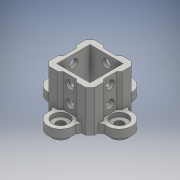
# Autodesk Inventor part: Mat_sup
Saved by Autodesk Inventor 2016 (Build 200138000, 138)
## iProperties
Created: 2016-07-08
Part Number: Mat_sup
Material: Générique
Document SubType Name: Modeling
Designer: LogOut
Density: 1 g/cm^3
Appearance: Par défaut
Author: LogOut
Autodesk Inventor part; units mm, degrees
ref_plane "YZ Plane" through (0, 0, 0) normal (1, 0, 0) x (0, 1, 0)
ref_plane "XZ Plane" through (0, 0, 0) normal (0, 1, 0) x (-1, 0, 0)
sketch "Esquisse1" plane through (0, 0, 0) normal (0, 0, 1) x (1, 0, 0)
  line L0 (-14.142136, 0) -> (0, -14.142136)
  line L1 (0, -14.142136) -> (14.142136, 0)
  line L2 (14.142136, 0) -> (0, 14.142136)
  line L3 (0, 14.142136) -> (-14.142136, 0)
  line L4 (-14.142136, 0) -> (14.142136, 0) construction
  line L5 (0, 14.142136) -> (0, -14.142136) construction
  line L6 (-20.142136, -20.142136) -> (20.142136, -20.142136)
  line L7 (20.142136, -20.142136) -> (20.142136, 20.142136)
  line L8 (20.142136, 20.142136) -> (-20.142136, 20.142136)
  line L9 (-20.142136, 20.142136) -> (-20.142136, -20.142136)
  circle A0 centre (14.142136, 0) radius 6
  circle A1 centre (0, -14.142136) radius 6
  circle A2 centre (-14.142136, 0) radius 6
  circle A3 centre (0, 14.142136) radius 6
  line L10 (0, 19.79899) -> (19.79899, 0)
  line L11 (19.79899, 0) -> (0, -19.79899)
  line L12 (0, -19.79899) -> (-19.79899, 0)
  line L13 (-19.79899, 0) -> (0, 19.79899)
  point P0 (0, 0)
  dimension "d4" = 20
  dimension "d5" = 20
  dimension "d10" = 6
  dimension "d11" = 6
  dimension "d12" = 6
  dimension "d13" = 6
  dimension "d19" = 4
  constraints: 28 end point, 6 parallel, 4 centre point, 4 coincident, 4 tangent, 3 perpendicular, 2 horizontal, 2 midpoint, 3 other
  measures "d4" distance between parallel lines of L0 L2
  measures "d5" distance between parallel lines of L1 L3
  measures "d10" distance from line of L8 L2.end
  measures "d11" distance from line of L9 L0.start
  measures "d12" distance from line of L7 L1.end
  measures "d13" distance from line of L0.end L6
  measures "d19" distance between parallel lines of L2 L10
extrude "Extrusion1" add sketch "Esquisse1" along normal blind 6 contours L3 A2 L0 | L0 A2 L12 L13 L3 | A2 L3 A3 L2 A0 L1 A1 L0 | L0 A1 L12 A2 | A2 L13 A3 L3 | A1 L1 L0 | L0 L1 A1 L11 L12 | A2 L13 L12 | A3 L13 L10 L2 L3 | L3 L2 A3 | L1 A0 L11 A1 | L12 L11 A1 | A3 L10 L13 | A3 L10 A0 L2 | A0 L2 L1 | L1 L2 A0 L10 L11 | L11 L10 A0
sketch "Esquisse2" plane through (0, 0, 0) normal (0, 0, -1) x (-1, 0, 0)
  line L0 (2.828427, 11.313708) -> (11.313708, 2.828427)
  arc A0 (4.242641, 9.899495) -> (-4.242641, 9.899495) centre (0, 14.142136) ccw
  line L1 (-11.313708, 2.828427) -> (-2.828427, 11.313708)
  arc A1 (-9.899495, 4.242641) -> (-9.899495, -4.242641) centre (-14.142136, 0) ccw
  line L2 (-2.828427, -11.313708) -> (-11.313708, -2.828427)
  arc A2 (-4.242641, -9.899495) -> (4.242641, -9.899495) centre (0, -14.142136) ccw
  line L3 (11.313709, -2.828427) -> (2.828427, -11.313708)
  arc A3 (9.899495, -4.242641) -> (9.899495, 4.242641) centre (14.142136, 0) ccw
  circle A4 centre (0, -14.142136) radius 4
  line L4 (-1.035276, -10.278432) -> (-10.278432, -1.035276)
  circle A5 centre (-14.142136, 0) radius 4
  line L5 (-10.278432, 1.035276) -> (-1.035276, 10.278432)
  circle A6 centre (0, 14.142136) radius 4
  line L6 (1.035276, 10.278432) -> (10.278432, 1.035276)
  circle A7 centre (14.142136, 0) radius 4
  line L7 (10.278432, -1.035276) -> (1.035276, -10.278432)
  line L8 (5.795555, -12.589221) -> (12.589221, -5.795555)
  line L9 (-12.589221, -5.795555) -> (-5.795555, -12.589221)
  line L10 (12.589221, 5.795555) -> (5.795555, 12.589221)
  line L11 (-5.795555, 12.589221) -> (-12.589221, 5.795555)
  line L12 (5.990705, -13.808285) -> (13.808285, -5.990705)
  line L13 (-13.808285, -5.990705) -> (-5.990705, -13.808285)
  line L14 (-5.990705, 13.808285) -> (-13.808285, 5.990705)
  line L15 (13.808285, 5.990705) -> (5.990705, 13.808285)
  point P0 (0, 0)
  dimension "d16" = 2
  constraints: 40 point on circle, 32 end point, 11 centre point, 8 point on line
  measures "d16" radial gap between concentric circles of A2 A4
extrude "Extrusion2" cut sketch "Esquisse2" against normal blind 2 contours A6 L1 A0 L0 | L0 A7 L6 A6 | A0 L10 A3 L0 | L6 A7 L7 A4 L4 A5 L5 A6 | A3 L3 A7 L0 | A0 L15 A3 L10 | L5 A5 L1 A6 | A7 L3 A4 L7 | L1 A1 L11 A0 | A0 L11 A1 L14 | A5 L2 A1 L1 | L12 A2 L8 A3 | L4 A4 L2 A5 | A3 L8 A2 L3 | L3 A2 L2 A4 | A1 L9 A2 L13 | L2 A2 L9 A1
sketch "Esquisse3" plane through (0, 0, 6) normal (0, 0, 1) x (1, 0, 0)
  line L0 (-5.990705, 13.808285) -> (-13.808285, 5.990705)
  arc A0 (-13.808285, 5.990705) -> (-13.808285, -5.990705) centre (-14.142136, 0) ccw
  line L1 (-13.808285, -5.990705) -> (-5.990705, -13.808285)
  arc A1 (-5.990705, -13.808285) -> (5.990705, -13.808285) centre (0, -14.142136) ccw
  line L2 (5.990705, -13.808285) -> (13.808285, -5.990705)
  arc A2 (13.808285, -5.990705) -> (13.808285, 5.990705) centre (14.142136, 0) ccw
  line L3 (13.808285, 5.990705) -> (5.990705, 13.808285)
  arc A3 (5.990705, 13.808285) -> (-5.990705, 13.808285) centre (0, 14.142136) ccw
  point P0 (0, 0)
hole "Perçage1" at (-14.142136, 0, 6) at (0, 14.142136, 6) at (14.142136, 0, 6) at (0, -14.142136, 6) direction (0, 0, -1) diameter 4 end through all counterbore diameter 8 counterbore depth 2
sketch "Esquisse4" plane through (0, 0, 6) normal (0, 0, 1) x (1, 0, 0)
  line L0 (-8, -8) -> (8, -8)
  line L1 (8, -8) -> (8, 8)
  line L2 (8, 8) -> (-8, 8)
  line L3 (-8, 8) -> (-8, -8)
  point P0 (0, 0)
  dimension "d27" = 8
  dimension "d28" = 8
  dimension "d29" = 16
  dimension "d33" = 16
  constraints: 8 end point, 2 parallel, 1 horizontal, 1 perpendicular
  measures "d27" distance from line of point (0, 0) L3
  measures "d28" distance from line of point (0, 0) L2
  measures "d29" distance between parallel lines of L3 L1
  measures "d33" distance between parallel lines of L2 L0
extrude "Extrusion3" cut sketch "Esquisse4" against normal through all
sketch "Esquisse5" plane through (0, 0, 6) normal (0, 0, 1) x (1, 0, 0)
  line L0 (8, 8) -> (8, -8)
  line L1 (8, -8) -> (-8, -8)
  line L2 (-8, -8) -> (-8, 8)
  line L3 (-8, 8) -> (8, 8)
  line L4 (-5.990705, 13.808285) -> (-13.808285, 5.990705)
  line L5 (-13.808285, -5.990705) -> (-5.990705, -13.808285)
  line L6 (5.990705, -13.808285) -> (13.808285, -5.990705)
  line L7 (13.808285, 5.990705) -> (5.990705, 13.808285)
  line L8 (-5.990705, 13.808285) -> (-13.808285, 5.990705)
  line L9 (-13.808285, 5.990705) -> (-10.979858, 3.162278)
  arc A0 (-10.979858, -3.162278) -> (-10.979858, 3.162278) centre (-14.142136, 0) ccw
  line L10 (-13.808285, -5.990705) -> (-10.979858, -3.162278)
  line L11 (8, -8) -> (-8, 8) construction
  line L12 (8, 8) -> (-8, -8) construction
  arc A1 (-3.162278, 10.979858) -> (3.162278, 10.979858) centre (0, 14.142136) ccw
  arc A2 (3.162278, -10.979858) -> (-3.162278, -10.979858) centre (0, -14.142136) ccw
  arc A3 (10.979858, 3.162278) -> (10.979858, -3.162278) centre (14.142136, 0) ccw
  line L13 (-5.990705, 13.808285) -> (-3.162278, 10.979858)
  line L14 (5.990705, 13.808285) -> (3.162278, 10.979858)
  line L15 (13.808285, 5.990705) -> (10.979858, 3.162278)
  line L16 (5.990705, -13.808285) -> (3.162278, -10.979858)
  line L17 (-5.990705, -13.808285) -> (-3.162278, -10.979858)
  line L18 (13.808285, -5.990705) -> (10.979858, -3.162278)
  point P0 (0, 0)
  constraints: 36 end point, 8 point on circle, 8 tangent, 4 centre point, 3 symmetric about line, 2 perpendicular, 3 other
extrude "Extrusion4" add sketch "Esquisse5" along normal blind 16
chamfer "Chanfrein1" distance 4 angle 45 8 edges at (-13.8083, 5.9907, 14) (-5.9907, 13.8083, 14) (5.9907, 13.8083, 14) (13.8083, 5.9907, 14) (13.8083, -5.9907, 14) (5.9907, -13.8083, 14) (-5.9907, -13.8083, 14) (-13.8083, -5.9907, 14)
sketch "Esquisse6" plane through (3.162278, 10.979858, 22) normal (0, 1, 0) x (1, 0, 0)
  line L0 (-3.1625, 12) -> (-3.1625, 4)
  line L1 (0, 16) -> (0, 0)
  line L2 (-6.324555, 16) -> (-6.324555, 0)
  line L3 (0, 0) -> (-6.324555, 0)
  point P0 (-3.162278, 22)
  dimension "d39" = 3.1625
  dimension "d40" = 3.16206
  dimension "d41" = 8
  dimension "d42" = 4
  constraints: 2 end point, 1 vertical
  measures "d39" distance between parallel lines of L1 L0
  measures "d40" distance between parallel lines of L0 L2
  measures "d41" distance of L0.start L0.end
  measures "d42" distance from line of L0.end L3
hole "Perçage2" at (-0.000222, 10.979858, 18) at (-0.000222, 10.979858, 10) direction (0, -1, 0) diameter 4 end through all
ref_plane "Plan de construction1" through (8, 8, 6) normal (-0.7071068, 0.7071068, 0) x (0, 0, -1)
mirror "Symétrie1" about plane through (8, 8, 6) normal (-0.7071068, 0.7071068, 0) of "Perçage2"
sketch "Esquisse7" plane through (0, 0, 22) normal (0, 0, 1) x (1, 0, 0)
  line L0 (8, -8) -> (-8, -8)
  line L1 (-8, -8) -> (-8, 8)
  line L2 (-8, 8) -> (8, 8)
  line L3 (8, 8) -> (8, -8)
  line L4 (-10.979858, -8.819132) -> (-10.979858, -3.162278)
  line L5 (-10.979858, -8.819132) -> (-8.819132, -10.979858)
  line L6 (-3.162278, -10.979858) -> (-8.819132, -10.979858)
  arc A0 (3.162278, -10.979858) -> (-3.162278, -10.979858) centre (0, -14.142136) ccw
  line L7 (8.819132, -10.979858) -> (3.162278, -10.979858)
  line L8 (8.819132, -10.979858) -> (10.979858, -8.819132)
  line L9 (10.979858, -3.162278) -> (10.979858, -8.819132)
  arc A1 (10.979858, 3.162278) -> (10.979858, -3.162278) centre (14.142136, 0) ccw
  line L10 (10.979858, 8.819132) -> (10.979858, 3.162278)
  line L11 (10.979858, 8.819132) -> (8.819132, 10.979858)
  line L12 (3.162278, 10.979858) -> (8.819132, 10.979858)
  arc A2 (-3.162278, 10.979858) -> (3.162278, 10.979858) centre (0, 14.142136) ccw
  line L13 (-8.819132, 10.979858) -> (-3.162278, 10.979858)
  line L14 (-8.819132, 10.979858) -> (-10.979858, 8.819132)
  line L15 (-10.979858, 3.162278) -> (-10.979858, 8.819132)
  arc A3 (-10.979858, -3.162278) -> (-10.979858, 3.162278) centre (-14.142136, 0) ccw
  line L16 (-3.162278, -10.979858) -> (3.162278, -10.979858)
  line L17 (3.162278, -10.979858) -> (3.162278, -9.67)
  line L18 (3.162278, -9.67) -> (-3.162278, -9.67)
  line L19 (-3.162278, -9.67) -> (-3.162278, -10.979858)
  line L20 (-10.979858, -3.162278) -> (-9.67, -3.162278)
  line L21 (-9.67, -3.162278) -> (-9.67, 3.162278)
  line L22 (-9.67, 3.162278) -> (-10.979858, 3.162278)
  line L23 (-10.979858, 3.162278) -> (-10.979858, -3.162278)
  line L24 (-5.09902, 10.979858) -> (-3.162278, 10.979858)
  line L25 (-3.162278, 10.979858) -> (3.162278, 10.979858)
  line L26 (3.162278, 10.979858) -> (3.162278, 9.67)
  line L27 (3.162278, 9.67) -> (-3.162278, 9.67)
  line L28 (-3.162278, 9.67) -> (-3.162278, 10.979858)
  arc A4 (10.979858, 3.162278) -> (10.979858, -3.162278) centre (14.142136, 0) ccw
  line L29 (10.979858, -3.162278) -> (9.67, -3.162278)
  line L30 (9.67, -3.162278) -> (9.67, 3.162278)
  line L31 (9.67, 3.162278) -> (10.979858, 3.162278)
  line L32 (10.979858, 3.162278) -> (10.979858, -3.162278)
  point P0 (0, 0)
  constraints: 32 end point, 8 parallel, 4 horizontal, 4 perpendicular, 1 point on line
extrude "Extrusion5" cut sketch "Esquisse7" against normal up to surface (16 mm away) contours L23 A3 | A3 L21 L20 | A3 L22 L21 | L19 L18 A0 | A0 L16 | L18 L17 A0 | L25 A2 | A2 L27 L28 | L29 L30 A1 | A1 L32 | A2 L26 L27 | L30 L31 A1
chamfer "Chanfrein2" distance 1.309 angle 45 8 edges at (-3.1623, -10.9799, 14) (3.1623, -10.9799, 14) (10.9799, -3.1623, 14) (10.9799, 3.1623, 14) (3.1623, 10.9799, 14) (-3.1623, 10.9799, 14) (-10.9799, 3.1623, 14) (-10.9799, -3.1623, 14)
chamfer "Chanfrein3" distance 2 angle 45 8 edges at (5.099, -10.9799, 4) (-5.099, -10.9799, 4) (10.9799, 5.099, 4) (10.9799, -5.099, 4) (-10.9799, 5.099, 4) (-10.9799, -5.099, 4) (5.099, 10.9799, 4) (-5.099, 10.9799, 4)
